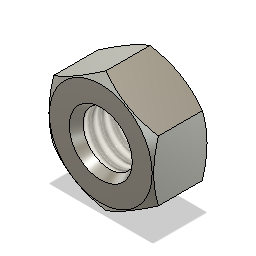
mechanism_v101 (Autodesk Fusion 360 archive; units mm, degrees)
design "Hexagon Regular Nut ISO 4032 - M6 Steel 6 Plain"
description: Hexagon Regular Nut ISO 4032 - M6
Autodesk Fusion 360 part; units mm, degrees
note: some values were not read from the file. Chosen so that the rebuilt part matches the saved one: which face or edge a step refers to; how an offset face is resized; the sign of a taper; which pieces of a blend or face edit are solid. Set by a fixed rule: which sketch regions a step uses.
sketch "Sketch1" plane through (0, 0, 0) normal (0, 1, 0) x (1, 0, 0)
  line L0 (0, 0) -> (0, -5.2)
  line L1 (-3, 0) -> (-4.9, 0)
  line L2 (-4.9, 0) -> (-5.775, -0.5052)
  line L3 (-5.775, -0.5052) -> (-5.775, -4.6948)
  line L4 (-5.775, -4.6948) -> (-4.9, -5.2)
  line L5 (-4.9, -5.2) -> (-3, -5.2)
  line L6 (-3, -5.2) -> (-3, 0)
  dimension "d121" = 6
  dimension "d122" = 30
  dimension "d123" = 30
  dimension "d126" = 5.2
  dimension "d128" = 11.55
  dimension "d172" = 9.8
  constraint vertical L0
  constraint coincident L0 L0.end
  constraint coincident origin L0
  constraint horizontal L1
  constraint perpendicular L1 L3
  constraint perpendicular L3 L5
  constraint perpendicular L5 L6
  constraint coincident L0.start L1
  constraint coincident L0.start origin
  constraint coincident L0.end L5
  constraint equal L1 L5
  measures "d122" angle of L1 L2
  measures "d123" angle of L4 L5
  measures "d126" distance of L1.start L5.end
revolve "Revolve1" add sketch "Sketch1" angle 360 about axis through (0, 0, 0) along (0, 0, 1)
sketch "Sketch8" plane through (0, 0, 5.2) normal (0, 0, 1) x (1, 0, 0)
  line L0 (0, 0) -> (-10, 0) construction
  line L1 (-5, -2.8897) -> (-5, 2.8897)
  circle A0 centre (0, 0) radius 3
  circle A1 centre (0, 0) radius 5.775
  dimension "d114" = 5
  constraint horizontal L0
  constraint perpendicular L0 L1
  constraint midpoint L0 L1
  constraint coincident L0.start A0.centre
  constraint coincident L1.end A1
  measures "d114" distance of L0.start L1
extrude "Extrude5" cut sketch "Sketch8" against normal blind 5.2 contours L1 A1 picked at (-5.125, -0.7039)
pattern_circular "C-Pattern2" count 6 over 360 about axis through (0, 0, 1.75) along (0, 0, 1) of "Extrude5"
thread "Thread3" "ISO Metric profile 6.0 M6x1 6H" major diameter 6.147 minor diameter 5.035 pitch 1 angle 60 resizes the face on face at (-2.9963, 0.1495, 3.4667)
sketch "Sketch12" plane through (0, 0, 0) normal (0, 1, 0) x (1, 0, 0)
  line L0 (2.5175, -5.2) -> (-2.5175, -5.2)
  line L1 (4.9, -5.2) -> (-4.9, -5.2)
  line L2 (4.9, 0) -> (-4.9, 0)
  line L3 (2.5175, 0) -> (-2.5175, 0)
  line L4 (-3, 0) -> (0, 0)
  line L5 (-1.4989, -2.6) -> (-3, 0)
  line L6 (-3, -5.2) -> (0, -5.2)
  line L7 (-1.4989, -2.6) -> (-3, -5.2)
  line L8 (0, 0) -> (0, -5.2)
  dimension "d165" = 60
  dimension "d169" = 60
  dimension "d170" = 3
  constraint horizontal L4
  constraint collinear L1 L6
  constraint coincident L5.start L7.start
  constraint vertical L4.start L6.start
  constraint coincident L1 L6.end
  constraint coincident L6.end L8.end
  constraint coincident L4.end L8.start
  measures "d165" angle of L2 L5
  measures "d169" angle of L6 L7
  measures "d170" distance of L4.start L4.end
revolve "Revolve3" cut sketch "Sketch12" angle 360 about axis through (0, 0, 1.75) along (0, 0, 1)
equation "adsk_nheig = 5.20 mm"
equation "adsk_maxdia = 11.55 mm"
equation "adsk_nomdia = 6.00 mm"
equation "d89 = -adsk_nheig"
equation "adsk_waflat = 10.00 mm"
equation "d114 = adsk_waflat / 2"
equation "adsk_chamang1 = 30.00 deg"
equation "adsk_chamang2 = 30.00 deg"
equation "d121 = adsk_nomdia"
equation "d122 = adsk_chamang1"
equation "d123 = adsk_chamang2"
equation "d126 = adsk_nheig"
equation "d128 = adsk_maxdia"
equation "d163 = adsk_nheig"
equation "d170 = adsk_nomdia * 0.5"
equation "adsk_beardia = adsk_waflat * 0.98"
equation "d172 = adsk_beardia"

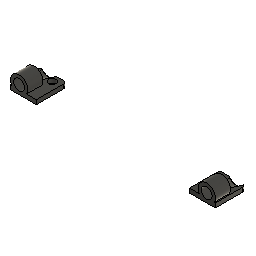
design "drzalo za kabel" references "Hexagon Socket Head Cap Screw ISO 4762 - M3 x 5 Steel 4.6 Plain"
Autodesk Fusion 360 part; units mm, degrees
sketch "Sketch3" plane through (0, 0, 0) normal (0, 0, 1) x (1, 0, 0)
  circle A0 centre (-8.4, 11) radius 1.75
  circle A1 centre (-8.4, 11) radius 2.9 construction
  line L0 (0, 0) -> (-12, 0)
  line L1 (-12, 0) -> (-12, 14)
  line L2 (-12, 14) -> (0, 14)
  line L3 (0, 14) -> (0, 0)
  dimension "d23" = 3.5
  dimension "d26" = 5.8
  dimension "d27" = 12
  dimension "d28" = 14
  dimension "d34" = 14
  dimension "d37" = 8.4
  constraint concentric A0 A1
  constraint vertical L1
  constraint horizontal L2
  constraint coincident L0.start L3.end
  measures "d23" diameter of A0
  measures "d26" diameter of A1
  measures "d27" distance of L0.start L0.end
  measures "d28" distance of L0.start L2.end
  measures "d34" distance of L0.end L1.end
  measures "d37" distance of A0.centre L3
extrude "Extrude4" add sketch "Sketch3" along normal blind 2 makes body 1
sketch "Sketch1" plane through (0, 0, 0) normal (0, 1, 0) x (1, 0, 0)
  line L0 (-3.5, 0.5) -> (-3.5, -2.1432) construction
  circle A0 centre (-4, -4) radius 2.5
  line L1 (-12, 0) -> (0, 0)
  line L2 (0, -2) -> (-12, -2)
  line L3 (-12, -2) -> (-12, 0)
  line L4 (0, 0) -> (-12, 0)
  line L5 (-12, 0) -> (-12, -2)
  line L6 (-12, -2) -> (0, -2)
  line L7 (0, -2) -> (0, 0)
  circle A1 centre (-4, -4) radius 4
  dimension "d6" = 5
  dimension "d33" = 4
  dimension "d36" = 8
  dimension "d38" = 4
  constraint vertical L0
  constraint concentric A0 A1
  measures "d6" diameter of A0
  measures "d33" distance of A0.centre L1
  measures "d36" diameter of A1
  measures "d38" distance of A0.centre L7
extrude "Extrude1" add sketch "Sketch1" along normal blind 7 contours A0 L2 L6 A1 | A0 L2 L6 A1 bodies 1
extrude "Extrude5" cut sketch "Sketch1" along normal through all contours A0 L2 L6 | A0 L2 L6 bodies 1
chamfer "Chamfer1" distance 1.5 distance2 2 1 edges at (-4, 14, 1.5) measured on face at (-9.8333, 14, 1.3333) on bodies 1
chamfer "Chamfer2" distance 2 angle 45 1 edges at (-4, 12, 1.5) on bodies 1
fillet "Fillet1" radius 1.5 2 edges at (-12, 14, 1) (0, 14, 1) on bodies 1
ref_plane "WorkPlane1" through (-47.5, 0, 0) normal (1, 0, 0) x (0, 1, 0)
mirror "Mirror1" about plane through (-47.5, 0, 0) normal (1, 0, 0) of bodies 1 makes body 2
other "Screw1"
component "drzalo za kabel v11" placed x (1, 0, 0) y (0, 1, 0) z (0, 0, 1) at (0, 0, 0)
equation "d36 = d33 * 2"
equation "d38 = d33"
equation "d44 = ( ( -95 / 2 ) * 1 mm )"
named bodies: "LL", "DD"

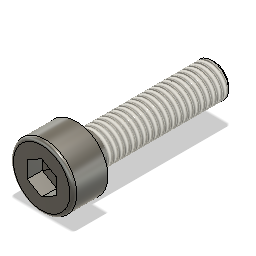
design "Hexagon Socket Head Cap Screw ISO 4762 - M3 x 12 Steel 4.6 Plain"
description: Hexagon Socket Head Cap Screw ISO 4762 - M3 x 12
part number: ISO 4762 - M3 x 12 Steel 4.6 Plain
Autodesk Fusion 360 part; units mm, degrees
sketch "Sketch1" plane through (0, 0, 0) normal (0, 1, 0) x (1, 0, 0)
  line L0 (-1.5, 0) -> (-1.5, 12)
  line L1 (-1.5, 12) -> (0, 12)
  line L2 (0, 12) -> (0, -3)
  line L3 (-1.5, 0) -> (-2.75, 0)
  line L4 (-2.75, 0) -> (-2.75, -3)
  line L5 (-2.75, -3) -> (0, -3)
  dimension "d9" = 3
  dimension "d66" = 5.5
  dimension "d106" = 3
  dimension "d107" = 12
  constraint perpendicular L0 L1
  constraint collinear origin L1.end L2.end
  constraint perpendicular L0 L3
  constraint coincident origin L3
  constraint vertical L0
  constraint vertical L2
  constraint parallel L2 L4
  constraint coincident L2 L5.end
  constraint perpendicular L2 L5
  measures "d106" distance of L3 L5
  measures "d107" distance of origin L1
revolve "Revolve1" add sketch "Sketch1" angle 360 about axis through (0, 0, -12) along (0, 0, 1)
ref_plane "WorkPlane1" through (0, 0, 3) normal (0, 0, 1) x (1, 0, 0)
sketch "Sketch6" plane through (0, 0, 3) normal (0, 0, 1) x (1, 0, 0)
  line L0 (-1.25, 0) -> (1.25, 0) construction
  line L1 (0, 0) -> (-1.25, 0.7217)
  line L2 (-1.25, -0.7217) -> (-1.25, 0.7217)
  line L3 (-1.25, -0.7217) -> (0, 0)
  dimension "d104" = 150
  dimension "d108" = 2.5
  constraint horizontal L0
  constraint midpoint L1.start L0
  constraint coincident L1.start L3.end
  constraint perpendicular L0 L2
  constraint midpoint L0.start L2
  constraint coincident L1.end L2.end
  measures "d104" angle of L0 L1
  measures "d108" distance of L0.end L2
extrude "Extrude1" cut sketch "Sketch6" against normal blind 1.3
pattern_circular "C-Pattern1" count 6 over 360 about axis through (0, 0, 1.75) along (0, 0, 1) of "Extrude1"
extrude "Extrude2" cut 1 faces at (0, 0.4811, 1.7) along direction (0, 0, -1) blind 1.3 draft -85
fillet "Fillet4" radius 0.3 1 edges at (-2.5639, 0.9944, 3)
thread "Thread2" "ISO Metric profile 3.0 M3x0.5 6g" major diameter 2.927 minor diameter 2.3555 pitch 0.5 angle 60 resizes the face on face at (-1.4925, 0.1494, -8)
sketch "Sketch7" plane through (0, 0, 0) normal (0, 1, 0) x (1, 0, 0)
  line L0 (-1.53, 12) -> (-1.53, 11.7)
  line L1 (-1.53, 11.7) -> (-1.23, 12)
  line L2 (0, 12) -> (0, -3)
  line L3 (-1.53, 12) -> (0, 12)
  dimension "d101" = 45
  dimension "d112" = 0.3
  dimension "d113" = 1.53
  constraint coincident L2.start L3.end
  constraint perpendicular L2 L3
  constraint coincident L1.end L3
  constraint perpendicular L0 L3
  measures "d101" angle of L0 L1
  measures "d112" distance of L0.end L3
  measures "d113" distance of L0 L2.start
revolve "Revolve3" cut sketch "Sketch7" angle 360 about axis through (0, 0, 1.75) along (0, 0, 1)
equation "d9 = adsk_nomdia"
equation "adsk_nomlen = 12.00 mm"
equation "adsk_headh = 3.00 mm"
equation "adsk_headdia = 5.50 mm"
equation "adsk_nomdia = 3.00 mm"
equation "adsk_philwidth = 2.50 mm"
equation "d31 = -adsk_phildepth"
equation "adsk_phildepth = 1.30 mm"
equation "d66 = adsk_headdia"
equation "d71 = adsk_headh"
equation "d76 = -adsk_phildepth"
equation "adsk_thrlen = 10.75 mm"
equation "d84 = adsk_thrlen"
equation "d86 = adsk_nomdia * 0.1"
equation "adsk_startang = 45.00 deg"
equation "d101 = adsk_startang"
equation "adsk_pitch1 = 0.50 mm"
equation "adsk_startlen = 0.30 mm"
equation "d106 = adsk_headh"
equation "d107 = adsk_nomlen"
equation "d108 = adsk_philwidth"
equation "d112 = adsk_startlen"
equation "d113 = adsk_nomdia * 0.51"

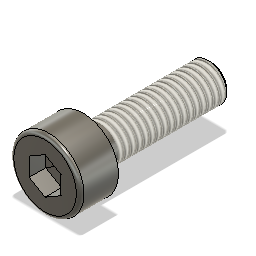
design "Hexagon Socket Head Cap Screw ISO 4762 - M3 x 10 Steel 4.6 Plain"
description: Hexagon Socket Head Cap Screw ISO 4762 - M3 x 10
Autodesk Fusion 360 part; units mm, degrees
sketch "Sketch1" plane through (0, 0, 0) normal (0, 1, 0) x (1, 0, 0)
  line L0 (-1.5, 0) -> (-1.5, 10)
  line L1 (-1.5, 10) -> (0, 10)
  line L2 (0, 10) -> (0, -3)
  line L3 (-1.5, 0) -> (-2.75, 0)
  line L4 (-2.75, 0) -> (-2.75, -3)
  line L5 (-2.75, -3) -> (0, -3)
  dimension "d9" = 3
  dimension "d66" = 5.5
  dimension "d68" = 10
  dimension "d79" = 3
  constraint perpendicular L0 L1
  constraint collinear origin L1.end L2.end
  constraint perpendicular L0 L3
  constraint coincident origin L3
  constraint vertical L0
  constraint vertical L2
  constraint parallel L2 L4
  constraint coincident L2 L5.end
  constraint perpendicular L2 L5
  measures "d68" distance of origin L1.end
  measures "d79" distance of L3.end L4.end
revolve "Revolve1" add sketch "Sketch1" angle 360 about axis through (0, 0, -10) along (0, 0, 1)
ref_plane "WorkPlane1" through (0, 0, 3) normal (0, 0, 1) x (1, 0, 0)
sketch "Sketch6" plane through (0, 0, 3) normal (0, 0, 1) x (1, 0, 0)
  line L0 (-1.25, 0) -> (1.25, 0) construction
  line L1 (0, 0) -> (-1.25, 0.7217)
  line L2 (-1.25, -0.7217) -> (-1.25, 0.7217)
  line L3 (-1.25, -0.7217) -> (0, 0)
  dimension "d72" = 2.5
  dimension "d104" = 150
  constraint horizontal L0
  constraint midpoint L1.start L0
  constraint coincident L1.start L3.end
  constraint perpendicular L0 L2
  constraint midpoint L0.start L2
  constraint coincident L1.end L2.end
  measures "d72" distance of L0.start L0.end
  measures "d104" angle of L0 L1
extrude "Extrude1" cut sketch "Sketch6" against normal blind 1.3
pattern_circular "C-Pattern1" count 6 over 360 about axis through (0, 0, 1.75) along (0, 0, 1) of "Extrude1"
extrude "Extrude2" cut 1 faces at (0, -0.4811, 1.7) along direction (0, 0, -1) blind 1.3 draft -85
fillet "Fillet4" radius 0.3 1 edges at (-2.5639, 0.9944, 3)
thread "Thread2" "ISO Metric profile 3.0 M3x0.5 6g" major diameter 2.927 minor diameter 2.3555 pitch 0.5 angle 60 resizes the face on face at (-1.4981, 0.0748, -3.3333)
sketch "Sketch7" plane through (0, 0, 0) normal (0, 1, 0) x (1, 0, 0)
  line L0 (-1.53, 10) -> (-1.53, 9.7)
  line L1 (-1.53, 9.7) -> (-1.23, 10)
  line L2 (0, 10) -> (0, -3)
  line L3 (-1.53, 10) -> (0, 10)
  dimension "d99" = 1.53
  dimension "d101" = 45
  dimension "d103" = 0.3
  constraint coincident L2.start L3.end
  constraint perpendicular L2 L3
  constraint coincident L1.end L3
  constraint perpendicular L0 L3
  measures "d99" distance of origin L0
  measures "d101" angle of L0 L1
  measures "d103" vertical distance of L0.end L1.end
revolve "Revolve3" cut sketch "Sketch7" angle 360 about axis through (0, 0, 1.75) along (0, 0, 1)
equation "d9 = adsk_nomdia"
equation "adsk_nomlen = 10.00 mm"
equation "adsk_headh = 3.00 mm"
equation "adsk_headdia = 5.50 mm"
equation "adsk_nomdia = 3.00 mm"
equation "adsk_philwidth = 2.50 mm"
equation "d31 = -adsk_phildepth"
equation "adsk_phildepth = 1.30 mm"
equation "d66 = adsk_headdia"
equation "d68 = adsk_nomlen"
equation "d71 = adsk_headh"
equation "d72 = adsk_philwidth"
equation "d76 = -adsk_phildepth"
equation "d79 = adsk_headh"
equation "adsk_thrlen = 8.75 mm"
equation "d84 = adsk_thrlen"
equation "d86 = adsk_nomdia * 0.1"
equation "d99 = adsk_nomdia * 0.51"
equation "adsk_startang = 45.00 deg"
equation "d101 = adsk_startang"
equation "adsk_pitch1 = 0.50 mm"
equation "d103 = adsk_startlen"
equation "adsk_startlen = 0.30 mm"

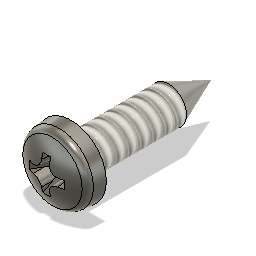
design "Type I Cross Recessed Pan Head Tapping Screw ANSI B18.6.5M 4.2x1.4 x 16 Type AB Steel Grade 2 Plain"
description: Type I Cross Recessed Pan Head Tapping Screw ANSI B18.6.5M 4.2x1.4 x 16 Type AB
Autodesk Fusion 360 part; units mm, degrees
sketch "Sketch1" plane through (0, 0, 0) normal (0, 1, 0) x (1, 0, 0)
  line L0 (-2.1, 0) -> (-2.1, 16)
  line L1 (-2.1, 16) -> (0, 16)
  line L2 (0, 16) -> (0, -3.1)
  line L3 (-2.1, 0) -> (-4, 0)
  line L4 (-4, 0) -> (-3.8385, -1.8455)
  arc A0 (-3.8385, -1.8455) -> (0, -3.1) centre (0, 3.4) ccw
  dimension "d9" = 4.2
  dimension "d66" = 8
  dimension "d67" = 3.1
  dimension "d68" = 16
  dimension "d70" = 6.5
  dimension "d92" = 85
  constraint perpendicular L0 L1
  constraint collinear origin L2.end L1.end
  constraint perpendicular L0 L3
  constraint coincident origin L3
  constraint vertical L0
  constraint vertical L2
  constraint coincident L2 A0.centre
  measures "d67" vertical distance of L2.end L3.end
  measures "d68" distance of origin L1.end
  measures "d70" radius of A0
  measures "d92" angle of L3 L4
revolve "Revolve1" add sketch "Sketch1" angle 360 about axis through (0, 0, -16) along (0, 0, 1) makes body 1
ref_plane "WorkPlane1" through (0, 0, 3.1) normal (0, 0, 1) x (1, 0, 0)
sketch "Sketch2" plane through (0, 0, 3.1) normal (0, 0, 1) x (1, 0, 0)
  circle A0 centre (0, 0) radius 3
  line L0 (-0.465, 2.2) -> (-0.465, 0.465)
  line L1 (-0.465, 0.465) -> (-2.2, 0.465)
  line L2 (0, 0) -> (0, 2.2) construction
  line L3 (0.465, 0.465) -> (2.2, 0.465)
  line L4 (0.465, 2.2) -> (0.465, 0.465)
  line L5 (0.465, -0.465) -> (2.2, -0.465)
  line L6 (0.465, -2.2) -> (0.465, -0.465)
  line L7 (-0.465, -2.2) -> (-0.465, -0.465)
  line L8 (-0.465, -0.465) -> (-2.2, -0.465)
  line L9 (-0.465, 2.2) -> (0.465, 2.2)
  line L10 (-2.2, 0.465) -> (-2.2, -0.465)
  line L11 (-0.465, -2.2) -> (0.465, -2.2)
  line L12 (2.2, -0.465) -> (2.2, 0.465)
  line L13 (1.75, 0) -> (22.5, 0)
  circle A1 centre (0, 0) radius 1.5
  dimension "d22" = 0.93
  dimension "d57" = 4.4
  constraint perpendicular L0 L1
  constraint coincident A0.centre L2.start
  constraint symmetric L0.start L2 L4.start
  constraint symmetric L0.end L2 L3.start
  constraint symmetric L1.end L2 L3.end
  constraint perpendicular L4 L9
  constraint perpendicular L8 L10
  constraint equal L9 L10
  constraint equal L0 L1
  constraint symmetric L1 L8 L13
  constraint horizontal L0.start L2.end
  constraint vertical L2
  constraint symmetric L3 L5 L13
  constraint symmetric L9 L11 L13
  constraint collinear L4 L6
  measures "d22" horizontal distance of L0.start L4.start
  measures "d57" distance of L10 L12
extrude "Extrude1" add sketch "Sketch2" against normal blind 2.45 draft -4 separate body contours L0 L4 L9 A1 | L0 L1 L3 L4 L5 L6 L7 L8 A1 | L1 L8 L10 A1 | L3 L5 L12 A1 | L6 L7 L11 A1 makes body 2
draft "Draft1" angle -30 neutral plane through (0, 0, 3.1) pull (0, 0, 1) 4 faces at (2.1429, -0.0979, 2.2833) (-0.0979, 2.1429, 2.2833) (-2.1429, -0.0979, 2.2833) (-0.0979, -2.1429, 2.2833) on bodies 2
fillet "Fillet3" radius 0.93 4 edges at (-0.3793, 0.3793, 1.875) (0.3793, 0.3793, 1.875) (0.3793, -0.3793, 1.875) (-0.3793, -0.3793, 1.875) on bodies 2
combine "Combine1" operation cut target body 1 tool bodies 2
fillet "Fillet5" radius 1.0333 1 edges at (-3.5788, 1.3881, 1.8455) on bodies 1
thread "Thread2" "Metric Forming Screw Threads 4.2 4.2x1.4 6g" major diameter 4.13 minor diameter 3.025 pitch 1.4 angle 60 resizes the face on face at (-2.0974, 0.1047, -5.3333) on bodies 1
sketch "Sketch5" plane through (0, 0, 0) normal (0, 1, 0) x (1, 0, 0)
  line L0 (-2.142, 10.9301) -> (0, 16)
  line L1 (-2.142, 16) -> (-2.142, 10.9301)
  line L2 (-2.142, 16) -> (0, 16)
  line L3 (0, 16) -> (0, -3.1)
  point P0 (0, 16)
  dimension "d90" = 5.0699
  dimension "d91" = 2.142
  constraint coincident L0.start L1.end
  constraint perpendicular L1 L2
  constraint coincident P0 L0.end
  constraint perpendicular L2 L3
  measures "d90" distance of L1.start L0.start
  measures "d91" horizontal distance of origin L1.start
revolve "Revolve2" cut sketch "Sketch5" angle 360 about axis through (0, 0, -16) along (0, 0, 1) bodies 1
equation "d9 = adsk_nomdia"
equation "adsk_nomlen = 16.00 mm"
equation "adsk_headh = 3.10 mm"
equation "adsk_headdia = 8.00 mm"
equation "adsk_nomdia = 4.20 mm"
equation "d22 = adsk_philwidth"
equation "adsk_phildia = 4.40 mm"
equation "d31 = -adsk_phildepth"
equation "adsk_philwidth = 0.93 mm"
equation "adsk_phildepth = 2.45 mm"
equation "d57 = adsk_phildia"
equation "d59 = adsk_philwidth"
equation "d66 = adsk_headdia"
equation "d67 = adsk_headh"
equation "d68 = adsk_nomlen"
equation "d70 = adsk_ovalrad"
equation "d71 = adsk_headh"
equation "adsk_startlen = 5.069855 mm"
equation "adsk_thrlen = 14.60 mm"
equation "d83 = adsk_headh / 3"
equation "d85 = adsk_thrlen"
equation "d90 = adsk_startlen"
equation "d91 = adsk_nomdia * 0.51"
equation "adsk_ovalrad = 6.50 mm"

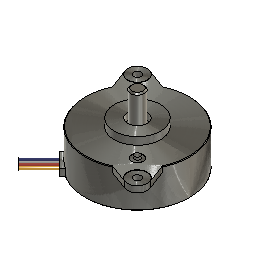
design "motor 12 mm"
Autodesk Fusion 360 part; units mm, degrees
sketch "Sketch1" plane through (0, 0, 0) normal (0, 0, 1) x (1, 0, 0)
  circle A0 centre (0, 0) radius 18
  line L0 (0, 0) -> (-12.9624, -12.9624)
  line L1 (0, 0) -> (18, 0) construction
  line L2 (-11.0178, -15.9676) -> (-15.9676, -11.0178)
  line L3 (-15.9676, -11.0178) -> (-14.9069, -9.9572)
  line L4 (-14.9069, -9.9572) -> (-9.9572, -14.9069) construction
  line L5 (-9.9572, -14.9069) -> (-11.0178, -15.9676)
  line L6 (-11.0178, -15.9676) -> (-14.9069, -9.9572) construction
  line L7 (-15.9676, -11.0178) -> (-9.9572, -14.9069) construction
  point P0 (-12.9624, -12.9624)
  dimension "d1" = 36
  dimension "d24" = 225
  dimension "d27" = 1.5
  dimension "d28" = 7
  constraint coincident A0.centre L0.start
  constraint horizontal L1
  constraint perpendicular L2 L3
  constraint parallel L2 L4
  constraint parallel L3 L5
  constraint coincident L6 P0
  constraint coincident L7 P0
  constraint coincident P0 L0.end
  constraint parallel L0 L3
  measures "d1" diameter of A0
  measures "d27" distance of L2.end L3.end
  measures "d28" distance of L3.end L4.end
extrude "Extrude1" add sketch "Sketch1" along normal blind 12.5 contours A0 makes body 1
extrude "Extrude5" add sketch "Sketch1" along normal blind 2.5 contours A0 L2 L3 L5 bodies 1
sketch "Sketch4" plane through (-13.4927, -13.4927, 0) normal (-0.707107, -0.707107, 0) x (0.707107, -0.707107, 0)
  line L0 (-3.5, 0) -> (3.5, 0)
  line L1 (3.5, 0) -> (3.5, 2.5)
  line L2 (3.5, 2.5) -> (-3.5, 2.5)
  line L3 (-3.5, 2.5) -> (-3.5, 0)
  circle A0 centre (-1.7487, 1.25) radius 0.5
  circle A1 centre (-0.5821, 1.25) radius 0.5
  circle A2 centre (0.5846, 1.25) radius 0.5
  circle A3 centre (1.7513, 1.25) radius 0.5
  dimension "d43" = 1
  dimension "d46" = 3.5
  dimension "d47" = 0
  measures "d43" diameter of A0
extrude "Extrude8" add sketch "Sketch4" along normal blind 10 separate body contours A0 | A1 | A2 | A3 makes body 2 at (-18.5744, -17.8391, 1.7461) makes body 3 at (-18.0273, -18.3862, 0.8751) makes body 4 at (-19.6772, -16.7363, 0.8751) makes body 5 at (-16.9244, -19.489, 1.7461)
sketch "Sketch2" plane through (0, 0, 12.5) normal (0, 0, 1) x (-1, 0, 0)
  circle A0 centre (0, 0) radius 18
  line L0 (-18.0003, 18.0003) -> (18.0003, -18.0003) construction
  line L1 (18.0001, 18.0001) -> (-21.5523, -21.5523) construction
  circle A1 centre (15.498, -15.498) radius 1.3
  arc A2 (-18, 0) -> (0, -18) centre (0, 0) ccw
  arc A3 (17.9997, 0.1002) -> (-0.1002, 17.9997) centre (0, 0) ccw
  circle A4 centre (15.498, -15.498) radius 3.4
  line L2 (18.6841, -14.3111) -> (16.2426, -7.7574)
  line L3 (14.3111, -18.6841) -> (7.7574, -16.2426)
  circle A5 centre (-15.498, 15.498) radius 1.3
  circle A6 centre (-15.498, 15.498) radius 3.4
  line L4 (-14.3111, 18.6841) -> (-7.7574, 16.2426)
  line L5 (-18.6841, 14.3111) -> (-16.2426, 7.7574)
  line L6 (0, 0) -> (13.513, 0) construction
  circle A7 centre (9.5459, -9.5459) radius 0.95
  circle A8 centre (9.5459, -9.5459) radius 2
  circle A9 centre (-9.5459, 9.5459) radius 0.95
  circle A10 centre (-9.5459, 9.5459) radius 2
  point P0 (15.498, -15.498)
  dimension "d6" = 21.9175
  dimension "d8" = 2.6
  dimension "d29" = 6.8
  dimension "d30" = 12
  dimension "d31" = 45
  dimension "d34" = 1.9
  dimension "d35" = 4
  dimension "d38" = 13.5
  constraint coincident L0 A0.centre
  constraint coincident L1 A0.centre
  constraint coincident A0.centre A2.centre
  constraint coincident L0 P0
  constraint coincident P0 A1.centre
  constraint coincident A4 L2.start
  constraint coincident A0 L2.end
  constraint symmetric L0 L2.start L3.start
  constraint symmetric L0 L2.end L3.end
  constraint symmetric L1 A1 A5
  constraint symmetric L1 A4 A6
  constraint symmetric L1 L2.start L4.start
  constraint symmetric L1 L2.end L4.end
  constraint symmetric L1 L3.start L5.start
  constraint symmetric L1 L3.end L5.end
  constraint horizontal L6
  constraint tangent A4 L2
  constraint perpendicular L0 L1
  constraint coincident L0 A7.centre
  constraint concentric A7 A8
  constraint symmetric L1 A7 A9
  constraint symmetric L1 A8 A10
  measures "d6" distance of A0.centre A1.centre
  measures "d8" diameter of A1
  measures "d29" diameter of A4
  measures "d30" distance of L2.end L3.end
  measures "d31" angle of L0 L6
  measures "d34" diameter of A7
  measures "d35" diameter of A8
  measures "d38" distance of A0.centre A7.centre
extrude "Extrude2" add sketch "Sketch2" against normal blind 2 contours A0 A2 A3 | A0 A4 L2 L3 | A4 | A0 A6 L4 L5 | A6 | A7 | A8 | A9 | A10 bodies 1
extrude "Extrude6" add sketch "Sketch2" along normal blind 0.1 contours A4 | A6 | A8 | A10 bodies 1
extrude "Extrude7" add sketch "Sketch2" along normal blind 1 contours A7 | A9 bodies 1
sketch "Sketch3" plane through (0, 0, 12.5) normal (0, 0, -1) x (-1, 0, 0)
  circle A0 centre (15.5563, 15.5563) radius 1.5
  circle A1 centre (0, 0) radius 2.375
  arc A2 (18.9879, 14.8678) -> (14.8678, 18.9879) centre (15.5563, 15.5563) ccw
  line L0 (14.8678, 18.9879) -> (7.021, 16.5743)
  line L1 (16.5743, 7.021) -> (18.9879, 14.8678)
  arc A3 (16.5743, 7.021) -> (7.021, 16.5743) centre (0, 0) ccw
  circle A4 centre (0, 0) radius 8
  arc A5 (-7.7574, -16.2426) -> (16.2426, 7.7574) centre (0, 0) ccw
  line L2 (-7.7574, -16.2426) -> (-14.3111, -18.6841)
  arc A6 (-14.3111, -18.6841) -> (-18.6841, -14.3111) centre (-15.498, -15.498) ccw
  line L3 (-18.6841, -14.3111) -> (-16.2426, -7.7574)
  arc A7 (7.7574, 16.2426) -> (-16.2426, -7.7574) centre (0, 0) ccw
  line L4 (7.7574, 16.2426) -> (14.3111, 18.6841)
  arc A8 (14.3111, 18.6841) -> (18.6841, 14.3111) centre (15.498, 15.498) ccw
  line L5 (18.6841, 14.3111) -> (16.2426, 7.7574)
  circle A9 centre (9.5459, 9.5459) radius 2
  circle A10 centre (-9.5459, -9.5459) radius 2
  circle A11 centre (0, 0) radius 3.35
  dimension "d12" = 4.75
  dimension "d21" = 16
  dimension "d39" = 6.7
  constraint coincident A1.centre A3.centre
  constraint concentric A3 A4
  constraint concentric A1 A11
  measures "d12" diameter of A1
  measures "d21" diameter of A4
  measures "d39" diameter of A11
extrude "Extrude4" add sketch "Sketch3" against normal blind 2.55 contours A4 bodies 1
extrude "Extrude3" add sketch "Sketch3" against normal blind 11.5 separate body contours A1 makes body 6
chamfer "Chamfer1" distance 0.5 angle 45 1 edges at (2.2143, 0.8588, 24) on bodies 6
fillet "Fillet1" radius 0.2 3 edges at (-12.7279, -12.7279, 12.5) (12.7279, 12.7279, 12.5) (12.7279, 12.7279, 0) on bodies 1
sketch "Sketch5" plane through (0, 0, 0) normal (0, 0, -1) x (1, 0, 0)
  line L0 (-15.9676, 11.0178) -> (-14.8157, 9.8659)
  arc A0 (-14.8157, 9.8659) -> (-9.8659, 14.8157) centre (0, 0) ccw
  line L1 (-9.8659, 14.8157) -> (-11.0178, 15.9676)
  line L2 (-11.0178, 15.9676) -> (-15.9676, 11.0178)
  line L3 (14.2464, 10.5632) -> (-10.7536, 10.5632) construction
  line L4 (-10.7536, 10.5632) -> (-10.7536, -10.4368) construction
  line L5 (-10.7536, -10.4368) -> (14.2464, -10.4368) construction
  line L6 (14.2464, -10.4368) -> (14.2464, 10.5632) construction
  dimension "d50" = 2
  text T0 "286230G\n\nSTH-36C0063\n\nSHINANO KENSHI" font "Arial" height 2 align centre middle in box 25 x 21 at (14.2464, 10.5632) x (-1, 0) y (0, -1) spacing 1
extrude "Extrude9" cut sketch "Sketch5" against normal blind 0.5 text T0 bodies 1
equation "d6 = ( ( 41.44 + 46.23 ) / 2 / 2 ) * 1 mm"
equation "d13 = -24 mm + 12.5 mm"
equation "d24 = 45 deg + 180 deg"
equation "d38 = ( ( 29 + 25 ) / 2 / 2 ) * 1 mm"

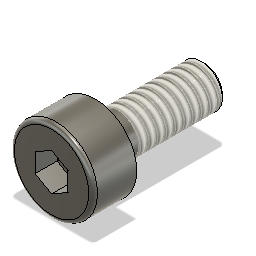
design "Hexagon Socket Head Cap Screw ISO 4762 - M2 x 5 Steel 4.6 Plain"
description: Hexagon Socket Head Cap Screw ISO 4762 - M2 x 5
Autodesk Fusion 360 part; units mm, degrees
sketch "Sketch1" plane through (0, 0, 0) normal (0, 1, 0) x (1, 0, 0)
  line L0 (-1, 0) -> (-1, 5)
  line L1 (-1, 5) -> (0, 5)
  line L2 (0, 5) -> (0, -2)
  line L3 (-1, 0) -> (-1.9, 0)
  line L4 (-1.9, 0) -> (-1.9, -2)
  line L5 (-1.9, -2) -> (0, -2)
  dimension "d9" = 2
  dimension "d66" = 3.8
  dimension "d68" = 5
  dimension "d79" = 2
  constraint perpendicular L0 L1
  constraint collinear origin L1.end L2.end
  constraint perpendicular L0 L3
  constraint coincident origin L3
  constraint vertical L0
  constraint vertical L2
  constraint parallel L2 L4
  constraint coincident L2 L5.end
  constraint perpendicular L2 L5
  measures "d68" distance of origin L1.end
  measures "d79" distance of L3.end L4.end
revolve "Revolve1" add sketch "Sketch1" angle 360 about axis through (0, 0, -5) along (0, 0, 1)
ref_plane "WorkPlane1" through (0, 0, 2) normal (0, 0, 1) x (1, 0, 0)
sketch "Sketch6" plane through (0, 0, 2) normal (0, 0, 1) x (1, 0, 0)
  line L0 (-0.75, 0) -> (0.75, 0) construction
  line L1 (0, 0) -> (-0.75, 0.433)
  line L2 (-0.75, -0.433) -> (-0.75, 0.433)
  line L3 (-0.75, -0.433) -> (0, 0)
  dimension "d72" = 1.5
  dimension "d104" = 150
  constraint horizontal L0
  constraint midpoint L1.start L0
  constraint coincident L1.start L3.end
  constraint perpendicular L0 L2
  constraint midpoint L0.start L2
  constraint coincident L1.end L2.end
  measures "d72" distance of L0.start L0.end
  measures "d104" angle of L0 L1
extrude "Extrude1" cut sketch "Sketch6" against normal blind 1
pattern_circular "C-Pattern1" count 6 over 360 about axis through (0, 0, 1.75) along (0, 0, 1) of "Extrude1"
extrude "Extrude2" cut 1 faces at (0, 0.2887, 1) along direction (0, 0, -1) blind 1 draft -85
fillet "Fillet4" radius 0.2 1 edges at (-1.7714, 0.6871, 2)
thread "Thread2" "ISO Metric profile 2.0 M2x0.4 6g" major diameter 1.9335 minor diameter 1.478 pitch 0.4 angle 60 resizes the face on face at (-0.995, 0.0996, -1.6667)
sketch "Sketch7" plane through (0, 0, 0) normal (0, 1, 0) x (1, 0, 0)
  line L0 (-1.02, 5) -> (-1.02, 4.8)
  line L1 (-1.02, 4.8) -> (-0.82, 5)
  line L2 (0, 5) -> (0, -2)
  line L3 (-1.02, 5) -> (0, 5)
  dimension "d99" = 1.02
  dimension "d101" = 45
  dimension "d103" = 0.2
  constraint coincident L2.start L3.end
  constraint perpendicular L2 L3
  constraint coincident L1.end L3
  constraint perpendicular L0 L3
  measures "d99" distance of origin L0
  measures "d101" angle of L0 L1
  measures "d103" vertical distance of L0.end L1.end
revolve "Revolve3" cut sketch "Sketch7" angle 360 about axis through (0, 0, 1.75) along (0, 0, 1)
equation "d9 = adsk_nomdia"
equation "adsk_nomlen = 5.00 mm"
equation "adsk_headh = 2.00 mm"
equation "adsk_headdia = 3.80 mm"
equation "adsk_nomdia = 2.00 mm"
equation "adsk_philwidth = 1.50 mm"
equation "d31 = -adsk_phildepth"
equation "adsk_phildepth = 1.00 mm"
equation "d66 = adsk_headdia"
equation "d68 = adsk_nomlen"
equation "d71 = adsk_headh"
equation "d72 = adsk_philwidth"
equation "d76 = -adsk_phildepth"
equation "d79 = adsk_headh"
equation "adsk_thrlen = 4.00 mm"
equation "d84 = adsk_thrlen"
equation "d86 = adsk_nomdia * 0.1"
equation "d99 = adsk_nomdia * 0.51"
equation "adsk_startang = 45.00 deg"
equation "d101 = adsk_startang"
equation "adsk_pitch1 = 0.40 mm"
equation "d103 = adsk_startlen"
equation "adsk_startlen = 0.20 mm"

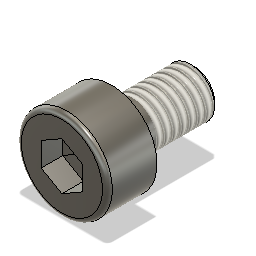
design "Hexagon Socket Head Cap Screw ISO 4762 - M3 x 5 Steel 4.6 Plain"
description: Hexagon Socket Head Cap Screw ISO 4762 - M3 x 5
part number: ISO 4762 - M3 x 5 Steel 4.6 Plain
Autodesk Fusion 360 part; units mm, degrees
sketch "Sketch1" plane through (0, 0, 0) normal (0, 1, 0) x (1, 0, 0)
  line L0 (-1.5, 0) -> (-1.5, 5)
  line L1 (-1.5, 5) -> (0, 5)
  line L2 (0, 5) -> (0, -3)
  line L3 (-1.5, 0) -> (-2.75, 0)
  line L4 (-2.75, 0) -> (-2.75, -3)
  line L5 (-2.75, -3) -> (0, -3)
  dimension "d9" = 3
  dimension "d66" = 5.5
  dimension "d106" = 3
  dimension "d107" = 5
  constraint perpendicular L0 L1
  constraint collinear origin L1.end L2.end
  constraint perpendicular L0 L3
  constraint coincident origin L3
  constraint vertical L0
  constraint vertical L2
  constraint parallel L2 L4
  constraint coincident L2 L5.end
  constraint perpendicular L2 L5
  measures "d106" distance of L3 L5
  measures "d107" distance of origin L1
revolve "Revolve1" add sketch "Sketch1" angle 360 about axis through (0, 0, -5) along (0, 0, 1)
ref_plane "WorkPlane1" through (0, 0, 3) normal (0, 0, 1) x (1, 0, 0)
sketch "Sketch6" plane through (0, 0, 3) normal (0, 0, 1) x (1, 0, 0)
  line L0 (-1.25, 0) -> (1.25, 0) construction
  line L1 (0, 0) -> (-1.25, 0.7217)
  line L2 (-1.25, -0.7217) -> (-1.25, 0.7217)
  line L3 (-1.25, -0.7217) -> (0, 0)
  dimension "d104" = 150
  dimension "d108" = 2.5
  constraint horizontal L0
  constraint midpoint L1.start L0
  constraint coincident L1.start L3.end
  constraint perpendicular L0 L2
  constraint midpoint L0.start L2
  constraint coincident L1.end L2.end
  measures "d104" angle of L0 L1
  measures "d108" distance of L0.end L2
extrude "Extrude1" cut sketch "Sketch6" against normal blind 1.3
pattern_circular "C-Pattern1" count 6 over 360 about axis through (0, 0, 1.75) along (0, 0, 1) of "Extrude1"
extrude "Extrude2" cut 1 faces at (0, -0.4811, 1.7) along direction (0, 0, -1) blind 1.3 draft -85
fillet "Fillet4" radius 0.3 1 edges at (-2.5639, 0.9944, 3)
thread "Thread2" "ISO Metric profile 3.0 M3x0.5 6g" major diameter 2.927 minor diameter 2.3555 pitch 0.5 angle 60 resizes the face on face at (-1.4981, 0.0748, -1.6667)
sketch "Sketch7" plane through (0, 0, 0) normal (0, 1, 0) x (1, 0, 0)
  line L0 (-1.53, 5) -> (-1.53, 4.7)
  line L1 (-1.53, 4.7) -> (-1.23, 5)
  line L2 (0, 5) -> (0, -3)
  line L3 (-1.53, 5) -> (0, 5)
  dimension "d101" = 45
  dimension "d112" = 0.3
  dimension "d113" = 1.53
  constraint coincident L2.start L3.end
  constraint perpendicular L2 L3
  constraint coincident L1.end L3
  constraint perpendicular L0 L3
  measures "d101" angle of L0 L1
  measures "d112" distance of L0.end L3
  measures "d113" distance of L0 L2.start
revolve "Revolve3" cut sketch "Sketch7" angle 360 about axis through (0, 0, 1.75) along (0, 0, 1)
equation "d9 = adsk_nomdia"
equation "adsk_nomlen = 5.00 mm"
equation "adsk_headh = 3.00 mm"
equation "adsk_headdia = 5.50 mm"
equation "adsk_nomdia = 3.00 mm"
equation "adsk_philwidth = 2.50 mm"
equation "d31 = -adsk_phildepth"
equation "adsk_phildepth = 1.30 mm"
equation "d66 = adsk_headdia"
equation "d71 = adsk_headh"
equation "d76 = -adsk_phildepth"
equation "adsk_thrlen = 3.75 mm"
equation "d84 = adsk_thrlen"
equation "d86 = adsk_nomdia * 0.1"
equation "adsk_startang = 45.00 deg"
equation "d101 = adsk_startang"
equation "adsk_pitch1 = 0.50 mm"
equation "adsk_startlen = 0.30 mm"
equation "d106 = adsk_headh"
equation "d107 = adsk_nomlen"
equation "d108 = adsk_philwidth"
equation "d112 = adsk_startlen"
equation "d113 = adsk_nomdia * 0.51"

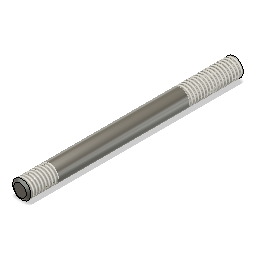
design "Double End Stud DIN 835 - M6 x 1 x 60 Steel 4.6 Plain"
description: Double End Stud DIN 835 - M6 x 1 x 60
Autodesk Fusion 360 part; units mm, degrees
sketch "Sketch1" plane through (0, 0, 0) normal (1, 0, 0) x (0, 0, -1)
  line L0 (60, 0) -> (-9.5, 0)
  line L1 (-9.5, 0) -> (-9.5, 3)
  line L2 (-9.5, 3) -> (60, 3)
  line L3 (60, 3) -> (60, 0)
  dimension "d1" = 6
  dimension "d54" = 9.5
  dimension "d55" = 60
  constraint horizontal L0
  constraint vertical L1
  constraint horizontal L2
  constraint vertical L3
  constraint coincident origin L0
  measures "d54" distance of origin L1
  measures "d55" distance of origin L3
revolve "Revolve1" add sketch "Sketch1" angle 360 about axis through (0, 0, -60) along (0, 0, 1)
thread "Thread3" "ISO Metric profile 6.0 M6x1 6g" major diameter 5.884 minor diameter 4.7435 pitch 1 angle 60 resizes the face on face at (0.1495, 2.9963, -13.6667)
thread "Thread4" "ISO Metric profile 6.0 M6x1 6g" thread offset 0 thread length 18
sketch "Sketch2" plane through (0, 0, 0) normal (1, 0, 0) x (0, 1, 0)
  line L0 (0, 9.5) -> (0, -60)
  line L1 (0, 9.5) -> (3.06, 9.5)
  line L2 (3.06, 9.5) -> (3.06, 8.8866)
  line L3 (3.06, 8.8866) -> (2, 9.5)
  line L4 (0, -60) -> (3.06, -60)
  line L5 (3.06, -60) -> (3.06, -59.3865)
  line L6 (3.06, -59.3865) -> (2, -60)
  dimension "d44" = 0.6135
  dimension "d45" = 3.06
  dimension "d46" = 2
  dimension "d48" = 0.6135
  dimension "d49" = 2
  dimension "d50" = 3.06
  constraint coincident L0.start L1.start
  constraint perpendicular L0 L1
  constraint perpendicular L1 L2
  constraint coincident L1 L3.end
  constraint coincident L0.end L4.start
  constraint perpendicular L0 L4
  constraint perpendicular L4 L5
  constraint coincident L4 L6.end
  measures "d44" distance of L1.end L2.end
  measures "d45" horizontal distance of L1.end origin
  measures "d46" horizontal distance of L3.end origin
  measures "d48" distance of L4.end L5.end
  measures "d49" horizontal distance of origin L6.end
  measures "d50" horizontal distance of origin L4.end
revolve "Revolve3" cut sketch "Sketch2" angle 360 about axis through (0, 0, -60) along (0, 0, 1)
equation "d1 = adsk_nomdia"
equation "adsk_nomdia = 6.00 mm"
equation "adsk_nomlen = 60.00 mm"
equation "adsk_thrlen = 18.00 mm"
equation "adsk_thrlen2 = 9.50 mm"
equation "d33 = adsk_thrlen2"
equation "d35 = adsk_thrlen"
equation "d44 = adsk_startlen"
equation "d45 = adsk_nomdia * 0.51"
equation "d46 = adsk_endpointdia / 2"
equation "d48 = d44"
equation "d49 = d46"
equation "d50 = d45"
equation "adsk_startlen = 0.61345 mm"
equation "adsk_endpointdia = 4.00 mm"
equation "d54 = adsk_thrlen2"
equation "d55 = adsk_nomlen"

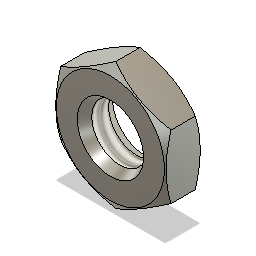
design "Hexagon Thin Nut ISO 4035 - M6 Steel 6 Plain"
description: Hexagon Thin Nut ISO 4035 - M6
Autodesk Fusion 360 part; units mm, degrees
sketch "Sketch1" plane through (0, 0, 0) normal (0, 1, 0) x (1, 0, 0)
  line L0 (0, 0) -> (0, -3.2)
  line L1 (-3, 0) -> (-4.9, 0)
  line L2 (-4.9, 0) -> (-5.775, -0.5052)
  line L3 (-5.775, -0.5052) -> (-5.775, -2.6948)
  line L4 (-5.775, -2.6948) -> (-4.9, -3.2)
  line L5 (-4.9, -3.2) -> (-3, -3.2)
  line L6 (-3, -3.2) -> (-3, 0)
  dimension "d121" = 6
  dimension "d122" = 30
  dimension "d123" = 30
  dimension "d126" = 3.2
  dimension "d128" = 11.55
  dimension "d172" = 9.8
  constraint vertical L0
  constraint coincident L0 L0.end
  constraint coincident origin L0
  constraint horizontal L1
  constraint perpendicular L1 L3
  constraint perpendicular L3 L5
  constraint perpendicular L5 L6
  constraint coincident L0.start L1
  constraint coincident L0.start origin
  constraint coincident L0.end L5
  constraint equal L1 L5
  measures "d122" angle of L1 L2
  measures "d123" angle of L4 L5
  measures "d126" distance of L1.start L5.end
revolve "Revolve1" add sketch "Sketch1" angle 360 about axis through (0, 0, 0) along (0, 0, 1)
sketch "Sketch8" plane through (0, 0, 3.2) normal (0, 0, 1) x (1, 0, 0)
  line L0 (0, 0) -> (-10, 0) construction
  line L1 (-5, -2.8897) -> (-5, 2.8897)
  circle A0 centre (0, 0) radius 3
  circle A1 centre (0, 0) radius 5.775
  dimension "d114" = 5
  constraint horizontal L0
  constraint perpendicular L0 L1
  constraint midpoint L0 L1
  constraint coincident L0.start A0.centre
  constraint coincident L1.end A1
  measures "d114" distance of L0.start L1
extrude "Extrude5" cut sketch "Sketch8" against normal blind 3.2 contours L1 A1 picked at (-5.125, -0.7039)
pattern_circular "C-Pattern2" count 6 over 360 about axis through (0, 0, 1.75) along (0, 0, 1) of "Extrude5"
thread "Thread3" "ISO Metric profile 6.0 M6x1 6H" major diameter 6.147 minor diameter 5.035 pitch 1 angle 60 resizes the face on face at (-2.9963, 0.1495, 2.1333)
sketch "Sketch12" plane through (0, 0, 0) normal (0, 1, 0) x (1, 0, 0)
  line L0 (2.5175, -3.2) -> (-2.5175, -3.2)
  line L1 (4.9, -3.2) -> (-4.9, -3.2)
  line L2 (4.9, 0) -> (-4.9, 0)
  line L3 (2.5175, 0) -> (-2.5175, 0)
  line L4 (-3, 0) -> (0, 0)
  line L5 (-2.0762, -1.6) -> (-3, 0)
  line L6 (-3, -3.2) -> (0, -3.2)
  line L7 (-2.0762, -1.6) -> (-3, -3.2)
  line L8 (0, 0) -> (0, -3.2)
  dimension "d165" = 60
  dimension "d169" = 60
  dimension "d170" = 3
  constraint horizontal L4
  constraint collinear L1 L6
  constraint coincident L5.start L7.start
  constraint vertical L4.start L6.start
  constraint coincident L1 L6.end
  constraint coincident L6.end L8.end
  constraint coincident L4.end L8.start
  measures "d165" angle of L2 L5
  measures "d169" angle of L6 L7
  measures "d170" distance of L4.start L4.end
revolve "Revolve3" cut sketch "Sketch12" angle 360 about axis through (0, 0, 1.75) along (0, 0, 1)
equation "adsk_nheig = 3.20 mm"
equation "adsk_maxdia = 11.55 mm"
equation "adsk_nomdia = 6.00 mm"
equation "d89 = -adsk_nheig"
equation "adsk_waflat = 10.00 mm"
equation "d114 = adsk_waflat / 2"
equation "adsk_chamang1 = 30.00 deg"
equation "adsk_chamang2 = 30.00 deg"
equation "d121 = adsk_nomdia"
equation "d122 = adsk_chamang1"
equation "d123 = adsk_chamang2"
equation "d126 = adsk_nheig"
equation "d128 = adsk_maxdia"
equation "d163 = adsk_nheig"
equation "d170 = adsk_nomdia * 0.5"
equation "adsk_beardia = adsk_waflat * 0.98"
equation "d172 = adsk_beardia"

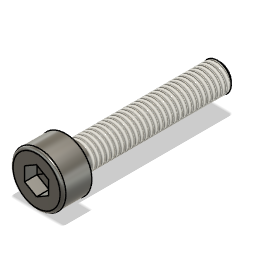
design "Hexagon Socket Head Cap Screw ISO 4762 - M3 x 16 Steel 4.6 Plain"
description: Hexagon Socket Head Cap Screw ISO 4762 - M3 x 16
part number: ISO 4762 - M3 x 16 Steel 4.6 Plain
Autodesk Fusion 360 part; units mm, degrees
sketch "Sketch1" plane through (0, 0, 0) normal (0, 1, 0) x (1, 0, 0)
  line L0 (-1.5, 0) -> (-1.5, 16)
  line L1 (-1.5, 16) -> (0, 16)
  line L2 (0, 16) -> (0, -3)
  line L3 (-1.5, 0) -> (-2.75, 0)
  line L4 (-2.75, 0) -> (-2.75, -3)
  line L5 (-2.75, -3) -> (0, -3)
  dimension "d9" = 3
  dimension "d66" = 5.5
  dimension "d106" = 3
  dimension "d107" = 16
  constraint perpendicular L0 L1
  constraint collinear origin L1.end L2.end
  constraint perpendicular L0 L3
  constraint coincident origin L3
  constraint vertical L0
  constraint vertical L2
  constraint parallel L2 L4
  constraint coincident L2 L5.end
  constraint perpendicular L2 L5
  measures "d106" distance of L3 L5
  measures "d107" distance of origin L1
revolve "Revolve1" add sketch "Sketch1" angle 360 about axis through (0, 0, -16) along (0, 0, 1)
ref_plane "WorkPlane1" through (0, 0, 3) normal (0, 0, 1) x (1, 0, 0)
sketch "Sketch6" plane through (0, 0, 3) normal (0, 0, 1) x (1, 0, 0)
  line L0 (-1.25, 0) -> (1.25, 0) construction
  line L1 (0, 0) -> (-1.25, 0.7217)
  line L2 (-1.25, -0.7217) -> (-1.25, 0.7217)
  line L3 (-1.25, -0.7217) -> (0, 0)
  dimension "d104" = 150
  dimension "d108" = 2.5
  constraint horizontal L0
  constraint midpoint L1.start L0
  constraint coincident L1.start L3.end
  constraint perpendicular L0 L2
  constraint midpoint L0.start L2
  constraint coincident L1.end L2.end
  measures "d104" angle of L0 L1
  measures "d108" distance of L0.end L2
extrude "Extrude1" cut sketch "Sketch6" against normal blind 1.3
pattern_circular "C-Pattern1" count 6 over 360 about axis through (0, 0, 1.75) along (0, 0, 1) of "Extrude1"
extrude "Extrude2" cut 1 faces at (0, 0.4811, 1.7) along direction (0, 0, -1) blind 1.3 draft -85
fillet "Fillet4" radius 0.3 1 edges at (-2.5639, 0.9944, 3)
thread "Thread2" "ISO Metric profile 3.0 M3x0.5 6g" major diameter 2.927 minor diameter 2.3555 pitch 0.5 angle 60 resizes the face on face at (-1.4925, 0.1494, -10.6667)
sketch "Sketch7" plane through (0, 0, 0) normal (0, 1, 0) x (1, 0, 0)
  line L0 (-1.53, 16) -> (-1.53, 15.7)
  line L1 (-1.53, 15.7) -> (-1.23, 16)
  line L2 (0, 16) -> (0, -3)
  line L3 (-1.53, 16) -> (0, 16)
  dimension "d101" = 45
  dimension "d112" = 0.3
  dimension "d113" = 1.53
  constraint coincident L2.start L3.end
  constraint perpendicular L2 L3
  constraint coincident L1.end L3
  constraint perpendicular L0 L3
  measures "d101" angle of L0 L1
  measures "d112" distance of L0.end L3
  measures "d113" distance of L0 L2.start
revolve "Revolve3" cut sketch "Sketch7" angle 360 about axis through (0, 0, 1.75) along (0, 0, 1)
equation "d9 = adsk_nomdia"
equation "adsk_nomlen = 16.00 mm"
equation "adsk_headh = 3.00 mm"
equation "adsk_headdia = 5.50 mm"
equation "adsk_nomdia = 3.00 mm"
equation "adsk_philwidth = 2.50 mm"
equation "d31 = -adsk_phildepth"
equation "adsk_phildepth = 1.30 mm"
equation "d66 = adsk_headdia"
equation "d71 = adsk_headh"
equation "d76 = -adsk_phildepth"
equation "adsk_thrlen = 14.75 mm"
equation "d84 = adsk_thrlen"
equation "d86 = adsk_nomdia * 0.1"
equation "adsk_startang = 45.00 deg"
equation "d101 = adsk_startang"
equation "adsk_pitch1 = 0.50 mm"
equation "adsk_startlen = 0.30 mm"
equation "d106 = adsk_headh"
equation "d107 = adsk_nomlen"
equation "d108 = adsk_philwidth"
equation "d112 = adsk_startlen"
equation "d113 = adsk_nomdia * 0.51"
